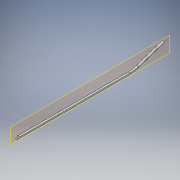
# Autodesk Inventor part: AAD0001149621
Saved by Autodesk Inventor 2017 (Build 210142000, 142)
## iProperties
Created: 2019-04-12
Part Number: AAD0001149621
Material: Generic
Document SubType Name: Modeling
Designer: Phs
Density: 1 g/cm^3
Appearance: Default
Author: Phs
Autodesk Inventor part; units mm, degrees
ref_plane "XZ Plane" through (0, 0, 0) normal (0, 1, 0) x (-1, 0, 0)
ref_plane "XY Plane" through (0, 0, 0) normal (0, 0, 1) x (1, 0, 0)
sketch "Sketch1" plane through (0, 0, 0) normal (0, 0, 1) x (1, 0, 0)
  line L0 (1, -23.75) -> (1, 25.75)
  line L1 (6, 30.75) -> (37, 30.75)
  line L2 (-37, -30.75) -> (-6, -30.75)
  arc A0 (-6, -30.75) -> (1, -23.75) centre (-6, -23.75) ccw
  arc A1 (6, 30.75) -> (1, 25.75) centre (6, 25.75) ccw
  line L3 (37, 32.75) -> (6, 32.75)
  arc A2 (6, 32.75) -> (-1, 25.75) centre (6, 25.75) ccw
  line L4 (-1, 25.75) -> (-1, -23.75)
  arc A3 (-6, -28.75) -> (-1, -23.75) centre (-6, -23.75) ccw
  line L5 (-6, -28.75) -> (-37, -28.75)
  line L6 (-37, -30.75) -> (-37, -28.75)
  line L7 (37, 30.75) -> (37, 32.75)
  point P0 (0, 0)
  dimension "d5" = 30.75
  dimension "d12" = 31
  dimension "d13" = 2
  constraints: 16 end point, 8 point on circle, 4 centre point, 3 parallel, 2 vertical, 1 horizontal, 4 other
  measures "d5" distance from line of point (0, 0) L1
  measures "d12" distance of L1.start L1.end
  measures "d13" distance between parallel lines of L0 L4
sketch "Sketch2" plane through (0, 0, 0) normal (1, 0, 0) x (0, 1, 0)
  line L0 (32.75, 0) -> (32.75, -1778.57)
  arc A0 (32.75, -1778.57) -> (55.2034, -1916.4389) centre (467.25, -1778.57) ccw
  line L1 (0, 0) -> (341.65, 0)
  line L2 (55.2034, -1916.4389) -> (194.6207, -2333.1133)
  dimension "d14" = 1778.57
  dimension "d17" = 161.5
  dimension "d18" = 439.38
  dimension "d28" = 434.5
  constraints: 6 end point, 2 point on circle, 2 tangent, 1 centre point, 1 horizontal, 1 vertical
  measures "d14" distance of L0.start L0.end
  measures "d17" angle of L2 L0
  measures "d18" distance of L2.start L2.end
  measures "d28" radius of A0
sweep "Sweep1" add profiles "Sketch1" path "Sketch2" path curves L0 A0 L2
sketch "Sketch3" plane through (1, -23.75, 0) normal (1, 0, 0) x (0, 0, -1)
  line L0 (0, 49.5) -> (0, 0) projected
  line L1 (0, 0) -> (1778.57, 0) projected
  arc A0 (1778.57, 0) -> (1934.3666, 25.3731) centre (1778.57, 491) ccw projected
  line L2 (1934.3666, 25.3731) -> (2351.041, 164.7904) projected
  line L3 (2335.3345, 211.7324) -> (2351.041, 164.7904) projected
  line L4 (1918.66, 72.3151) -> (2335.3345, 211.7324) projected
  arc A1 (1778.57, 49.5) -> (1918.66, 72.3151) centre (1778.57, 491) ccw projected
  line L5 (0, 49.5) -> (1778.57, 49.5) projected
  line L6 (50, 83.8551) -> (50, -57.0573)
  line L7 (458.25, 83.8551) -> (458.25, -57.0573)
  line L8 (653.5, 83.8551) -> (653.5, -57.0573)
  circle A2 centre (1778.57, 491) radius 467.25
  line L9 (2343.1877, 188.2614) -> (1927.8399, 48.2348)
  line L10 (2020.5284, 268.8859) -> (2149.5287, -116.6554)
  line L11 (1818.57, 100.4548) -> (1818.57, -125.8263)
  line L12 (1936.5877, 18.7348) -> (1934.3666, 25.3731) projected
  line L13 (1778.57, -7) -> (1778.57, 0) projected
  circle A3 centre (2077.4777, 98.6823) radius 10
  circle A4 centre (1818.57, 25.4653) radius 10
  circle A5 centre (653.5, 23.75) radius 10
  circle A6 centre (458.25, 23.75) radius 10
  circle A7 centre (50, 23.75) radius 10
  point P0 (0, 23.75)
  dimension "d22" = 408.25
  dimension "d23" = 195.25
  dimension "d24" = 40
  dimension "d26" = 158.977
  dimension "d29" = 20
  dimension "d30" = 20
  dimension "d31" = 20
  dimension "d32" = 20
  dimension "d33" = 20
  constraints: 12 end point, 6 centre point, 6 point on line, 2 parallel, 2 point on circle, 2 vertical, 1 coincident, 1 midpoint, 1 tangent
  measures "d22" distance between parallel lines of L7 L6
  measures "d23" distance between parallel lines of L8 L7
  measures "d24" distance from line of L11 L1.end
  measures "d26" distance between parallel lines of L10 L12
  measures "d29" diameter of A3
  measures "d30" diameter of A4
  measures "d31" diameter of A5
  measures "d32" diameter of A6
  measures "d33" diameter of A7
extrude "Extrusion1" cut sketch "Sketch3" against normal blind 10 contours A7 L6 | L6 A7 | A6 L7 | L7 A6 | A5 L8 | L8 A5 | A4 L11 A2 | A2 L11 A4 | L11 A4 A2 | A2 A4 L11 | A3 L9 L10 | L10 L9 A3 | A3 L9 L10 | L10 L9 A3
sketch "Sketch4" plane through (1, -23.75, 0) normal (1, 0, 0) x (0, 0, -1)
  line L0 (2335.3345, 211.7324) -> (2333.1133, 218.3707) projected
  line L1 (2333.1133, 218.3707) -> (2363.5204, -278.781)
  line L2 (1778.57, -7) -> (1778.57, 0) projected
  line L3 (2333.1133, 218.3707) -> (2448.2703, 211.7324)
  line L4 (2448.2703, 211.7324) -> (2363.5204, -278.781)
  point P0 (0, 23.75)
  dimension "d36" = 3.5
  constraints: 6 end point
  measures "d36" angle of L1 L2
extrude "Extrusion2" cut sketch "Sketch4" along normal through all both and the other way through all
body "Solid1"
